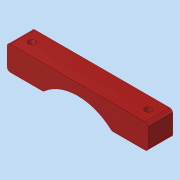
# Autodesk Inventor part: Top
Saved by Autodesk Inventor 2017.3 (Build 213256000, 256)
## iProperties
Created: 2018-07-27
Part Number: Top
Material: ABS Plastic
Document SubType Name: Modeling
Designer: Derek Wider
Density: 1.06 g/cm^3
Appearance: Red
Author: Derek Wider
Autodesk Inventor part; units mm, degrees
ref_plane "YZ Plane" through (0, 0, 0) normal (1, 0, 0) x (0, 1, 0)
ref_plane "XZ Plane" through (0, 0, 0) normal (0, 1, 0) x (-1, 0, 0)
ref_plane "XY Plane" through (0, 0, 0) normal (0, 0, 1) x (1, 0, 0)
sketch "Sketch1" plane through (0, 0, 0) normal (0, 0, 1) x (1, 0, 0)
  line L0 (-73.025, 0) -> (-73.025, 25.4)
  line L1 (-73.025, 25.4) -> (73.025, 25.4)
  line L2 (73.025, 25.4) -> (73.025, 0)
  line L3 (73.025, 0) -> (35.4919, 0)
  line L4 (-73.025, 0) -> (-35.4919, 0)
  arc A0 (35.4919, 0) -> (-35.4919, 0) centre (0, -38.1) ccw
  point P0 (0, 0)
  dimension "d1" = 104.14
  dimension "d2" = 38.1
  dimension "d3" = 146.05
  dimension "d4" = 25.4
  constraints: 10 end point, 3 perpendicular, 2 horizontal alignment, 2 point on circle, 1 centre point, 1 collinear, 1 horizontal, 1 vertical, 1 vertical alignment
  measures "d1" diameter of A0
  measures "d2" vertical distance of L4.end A0.centre
  measures "d3" distance of L0.end L1.end
  measures "d4" distance of L0.start L0.end
extrude "Extrusion1" add sketch "Sketch1" along normal blind 25.4
sketch "Sketch2" plane through (-73.025, 25.4, 0) normal (0, 1, 0) x (1, 0, 0)
  line L0 (0, 0) -> (146.05, 0) construction
  line L1 (0, 0) -> (0, -25.4) construction
  line L2 (146.05, -25.4) -> (0, -25.4) construction
  line L3 (146.05, 0) -> (146.05, -25.4) construction
  circle A0 centre (12.7, -12.7) radius 3.4925
  circle A1 centre (133.35, -12.7) radius 3.4925
  point P0 (73.025, 0)
  dimension "d7" = 6.985
  dimension "d8" = 6.985
  dimension "d9" = 12.7
  dimension "d10" = 12.7
  constraints: 2 centre point
  measures "d7" diameter of A0
  measures "d8" diameter of A1
  measures "d9" distance from line of A0.centre L1
  measures "d10" distance from line of A1.centre L3
extrude "Extrusion2" cut sketch "Sketch2" against normal through all
fillet "Fillet1" radius 3.175 6 edges at (73.025, 25.4, 12.7) (-73.025, 25.4, 12.7) (-73.025, 0, 12.7) (-35.4919, 0, 12.7) (35.4919, 0, 12.7) (73.025, 0, 12.7)
body "Solid1"
